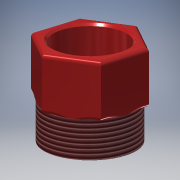
# Autodesk Inventor part: Component 33(Intake Pipe Union)
Saved by Autodesk Inventor 2018 (Build 220112000, 112)
## iProperties
Created: 2023-04-01
Part Number: Component 33(Intake Pipe Union)
Material: Generic
Document SubType Name: Modeling
Designer: Habib Mohamed
Density: 1 g/cm^3
Appearance: Light Red
Author: Habib Mohamed
Autodesk Inventor part; units mm, degrees
ref_plane "YZ Plane" through (0, 0, 0) normal (1, 0, 0) x (0, 1, 0)
ref_plane "XZ Plane" through (0, 0, 0) normal (0, 1, 0) x (-1, 0, 0)
ref_plane "XY Plane" through (0, 0, 0) normal (0, 0, 1) x (1, 0, 0)
sketch "Sketch1" plane through (0, 0, 0) normal (0, 1, 0) x (-1, 0, 0)
  circle A0 centre (0, 0) radius 5 construction
  line L0 (5, -2.886751) -> (0, -5.773503)
  line L1 (0, -5.773503) -> (-5, -2.886751)
  line L2 (-5, -2.886751) -> (-5, 2.886751)
  line L3 (-5, 2.886751) -> (0, 5.773503)
  line L4 (0, 5.773503) -> (5, 2.886751)
  line L5 (5, 2.886751) -> (5, -2.886751)
  point P0 (5, 0)
  dimension "d0" = 10
  constraints: 12 end point, 2 coincident, 1 horizontal alignment, 1 midpoint, 15 other
extrude "Extrusion1" add sketch "Sketch1" along normal blind 6
sketch "Sketch2" plane through (0, 0, 0) normal (0, -1, 0) x (1, 0, 0)
  circle A0 centre (0, 0) radius 5
  constraints: 1 centre point, 1 coincident
extrude "Extrusion2" add sketch "Sketch2" along normal blind 10 from surface at -6
sketch "Sketch3" plane through (0, 6, 0) normal (0, 1, 0) x (1, 0, 0)
  circle A0 centre (0, 0) radius 4
  dimension "d5" = 8
  constraints: 1 centre point, 1 coincident
  measures "d5" diameter of A0
extrude "Extrusion3" cut sketch "Sketch3" against normal through all
chamfer "Chamfer1" distance 0.25 angle 45 2 edges at (-4, -4, 0) (-4, 6, 0)
fillet "Fillet1" radius 0.5 6 edges at (-2.5, 6, 4.3301) (-5, 6, 0) (-2.5, 6, -4.3301) (2.5, 6, -4.3301) (5, 6, 0) (2.5, 6, 4.3301)
fillet "Fillet2" radius 0.5 12 edges at (-1.25, 0, 5.0518) (-3.75, 0, 3.6084) (-5, 0, 1.4434) (1.25, 0, 5.0518) (3.75, 0, 3.6084) (5, 0, 1.4434) (5, 0, -1.4434) (3.75, 0, -3.6084) (1.25, 0, -5.0518) (-1.25, 0, -5.0518) (-3.75, 0, -3.6084) (-5, 0, -1.4434)
thread "Thread1" size "M10x1" class "6g" standard "ANSI Metric M Profile" length 4
body "Solid1"
